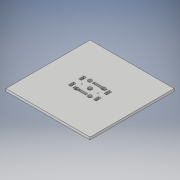
# Autodesk Inventor part: thumper-base-v2
Saved by Autodesk Inventor 2017 (Build 210142000, 142)
## iProperties
Created: 2017-02-22
Part Number: thumper-base-v2
Material: Generic
Document SubType Name: Modeling
Designer: John
Density: 1 g/cm^3
Appearance: Default
Author: John
Autodesk Inventor part; units mm, degrees
ref_plane "YZ Plane" through (0, 0, 0) normal (1, 0, 0) x (0, 1, 0)
ref_plane "XZ Plane" through (0, 0, 0) normal (0, 1, 0) x (-1, 0, 0)
ref_plane "XY Plane" through (0, 0, 0) normal (0, 0, 1) x (1, 0, 0)
sketch "Sketch1" plane through (0, 0, 0) normal (0, 1, 0) x (-1, 0, 0)
  point P0 (0, 0)
sketch "Sketch2" plane through (0, 0, 0) normal (0, 1, 0) x (-1, 0, 0)
  line L0 (-100, 100) -> (100, 100)
  line L1 (100, 100) -> (100, -100)
  line L2 (100, -100) -> (-100, -100)
  line L3 (-100, -100) -> (-100, 100)
  line L4 (-100, 100) -> (100, -100) construction
  line L5 (100, 100) -> (-100, -100) construction
  line L6 (27, -18.5) -> (33, -18.5)
  line L7 (33, -18.5) -> (33, -6.5)
  line L8 (33, -6.5) -> (27, -6.5)
  line L9 (27, -6.5) -> (27, -18.5)
  line L10 (27, -18.5) -> (33, -6.5) construction
  line L11 (33, -18.5) -> (27, -6.5) construction
  line L12 (0, 100) -> (0, -100) construction
  line L13 (100, 0) -> (-100, 0) construction
  circle A0 centre (0, 0) radius 5
  circle A1 centre (16, -16) radius 4.5
  circle A2 centre (-16, 16) radius 4.5
  line L14 (8, -13.5) -> (-22, -13.5)
  line L15 (-22, -13.5) -> (-22, -18.5)
  line L16 (-22, -18.5) -> (8, -18.5)
  line L17 (8, -18.5) -> (8, -13.5)
  line L18 (-8, 13.5) -> (22, 13.5)
  line L19 (22, 13.5) -> (22, 18.5)
  line L20 (22, 18.5) -> (-8, 18.5)
  line L21 (-8, 18.5) -> (-8, 13.5)
  circle A3 centre (18.9997, 0) radius 1
  circle A4 centre (-18.9997, 0) radius 1
  line L22 (27, 18.5) -> (33, 18.5)
  line L23 (33, 18.5) -> (33, 6.5)
  line L24 (33, 6.5) -> (27, 6.5)
  line L25 (27, 6.5) -> (27, 18.5)
  line L26 (27, 18.5) -> (33, 6.5) construction
  line L27 (33, 18.5) -> (27, 6.5) construction
  line L28 (-27, -18.5) -> (-33, -18.5)
  line L29 (-33, -18.5) -> (-33, -6.5)
  line L30 (-33, -6.5) -> (-27, -6.5)
  line L31 (-27, -6.5) -> (-27, -18.5)
  line L32 (-27, -18.5) -> (-33, -6.5) construction
  line L33 (-33, -18.5) -> (-27, -6.5) construction
  line L34 (-27, 6.5) -> (-27, 18.5)
  line L35 (-27, 18.5) -> (-33, 18.5)
  line L36 (-33, 18.5) -> (-33, 6.5)
  line L37 (-27, 18.5) -> (-33, 6.5) construction
  line L38 (-33, 18.5) -> (-27, 6.5) construction
  line L39 (-33, 6.5) -> (-27, 6.5)
  circle A5 centre (16, 16) radius 4.5
  circle A6 centre (-16, -16) radius 4.5
  point P0 (30, -12.5)
  point P1 (30, 12.5)
  point P2 (-30, -12.5)
  point P3 (-30, 12.5)
  dimension "d0" = 200
  dimension "d1" = 200
  dimension "d3" = 12
  dimension "d5" = 10
  dimension "d8" = 9
  dimension "d10" = 16
  dimension "d11" = 16
  dimension "d15" = 30
  dimension "d16" = 5
  dimension "d17" = 13.5
  dimension "d18" = 8
  dimension "d19" = 30
  dimension "d20" = 5
  dimension "d21" = 13.5
  dimension "d22" = 8
  dimension "d23" = 2
  dimension "d24" = 8.0003
  dimension "d27" = 6
  dimension "d30" = 30
  constraints: 80 end point, 19 symmetric about line, 14 midpoint, 8 parallel, 7 centre point, 4 horizontal, 4 perpendicular, 1 coincident, 1 collinear, 1 point on line, 4 other
  measures "d0" distance of L1.end L2.end
  measures "d1" distance of L0.end L1.end
  measures "d3" distance of L7.end L6.end
  measures "d5" diameter of A0
  measures "d8" diameter of A1
  measures "d10" horizontal distance of point (0, 0) A1.centre
  measures "d11" horizontal distance of A0.centre A1.centre
  measures "d15" distance of L16.end L15.end
  measures "d16" distance of L15.end L14.end
  measures "d17" distance from line of point (0, 0) L14
  measures "d18" distance between parallel lines of L17 L12
  measures "d19" distance of L20.end L19.end
  measures "d20" distance of L19.end L18.end
  measures "d21" distance between parallel lines of L13 L18
  measures "d22" distance between parallel lines of L21 L12
  measures "d23" diameter of A3
  measures "d24" distance from line of A3.centre L9
  measures "d27" distance of L7.end L8.end
  measures "d30" horizontal distance of point (0, 0) point (30, -12.5)
extrude "Extrusion1" add sketch "Sketch2" along normal blind 6
body "Solid1"
